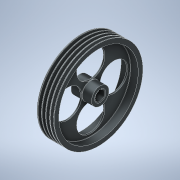
# Autodesk Inventor part: Polia Movida sem alivio de peso
Saved by Autodesk Inventor 2021 (Build 250183000, 183)
## iProperties
Created: 2021-03-22
Part Number: Polia Movida sem alivio de peso
Material: Iron, Cast
Document SubType Name: Modeling
Designer: mathe
Density: 7.15 g/cm^3
Appearance: Iron Gray
Mass: 8408.41 g
Surface Area: 3444.04 cm^2
Volume: 1176 cm^3
Author: mathe
Autodesk Inventor part; units mm, degrees
ref_plane "YZ Plane" through (0, 0, 0) normal (1, 0, 0) x (0, 1, 0)
ref_plane "XZ Plane" through (0, 0, 0) normal (0, 1, 0) x (-1, 0, 0)
ref_plane "XY Plane" through (0, 0, 0) normal (0, 0, 1) x (1, 0, 0)
sketch "Sketch1" plane through (0, 0, 0) normal (0, 0, 1) x (1, 0, 0)
  line L0 (68.9593, 13.1588) -> (64.9475, 24.81)
  line L1 (84.8393, 13.1588) -> (80.8275, 24.81)
  arc A0 (71.5582, 12.4844) -> (72.5037, 13.1588) centre (71.5582, 13.4844) ccw
  arc A1 (77.461, 25.4844) -> (76.5155, 24.81) centre (77.461, 24.4844) ccw
  line L2 (72.5037, 13.1588) -> (76.5155, 24.81)
  line L3 (56.6237, 13.1588) -> (60.6355, 24.81)
  arc A2 (82.7615, 30.4844) -> (83.7615, 31.4844) centre (82.7615, 31.4844) ccw
  arc A3 (82.7615, 30.4844) -> (83.7615, 31.4844) centre (82.7615, 31.4844) ccw
  arc A4 (80.8275, 24.81) -> (79.8819, 25.4844) centre (79.8819, 24.4844) ccw
  line L4 (69.9048, 12.4844) -> (71.5582, 12.4844)
  arc A5 (68.9593, 13.1588) -> (69.9048, 12.4844) centre (69.9048, 13.4844) ccw
  arc A6 (64.9475, 24.81) -> (64.0019, 25.4844) centre (64.0019, 24.4844) ccw
  line L5 (61.581, 25.4844) -> (64.0019, 25.4844)
  arc A7 (61.581, 25.4844) -> (60.6355, 24.81) centre (61.581, 24.4844) ccw
  arc A8 (55.6782, 12.4844) -> (56.6237, 13.1588) centre (55.6782, 13.4844) ccw
  line L6 (53.2615, 12.4844) -> (55.6782, 12.4844)
  line L7 (53.2615, 12.4844) -> (53.2615, 25.4844)
  line L8 (53.2615, 12.4844) -> (53.2615, 25.4844)
  line L9 (53.2615, 30.4844) -> (82.7615, 30.4844)
  line L10 (53.2615, 30.4844) -> (82.7615, 30.4844)
  line L11 (53.2615, 25.4844) -> (53.2615, 30.4844)
  line L12 (53.2615, 25.4844) -> (53.2615, 30.4844)
  line L13 (77.461, 25.4844) -> (79.8819, 25.4844)
  line L14 (83.7615, 149.9844) -> (83.7615, 31.4844)
  line L15 (89.7615, 149.9844) -> (89.7615, 31.4844)
  line L16 (83.7615, 149.9844) -> (83.7615, 31.4844)
  line L17 (89.7615, 149.9844) -> (89.7615, 31.4844)
  line L18 (68.9593, 356.81) -> (64.9475, 345.1588)
  line L19 (84.8393, 356.81) -> (80.8275, 345.1588)
  line L20 (88.3837, 356.81) -> (92.3955, 345.1588)
  arc A9 (72.5037, 356.81) -> (71.5582, 357.4844) centre (71.5582, 356.4844) ccw
  arc A10 (76.5155, 345.1588) -> (77.461, 344.4844) centre (77.461, 345.4844) ccw
  line L21 (53.2615, 339.4844) -> (82.7615, 339.4844)
  line L22 (53.2615, 339.4844) -> (82.7615, 339.4844)
  arc A11 (69.9048, 357.4844) -> (68.9593, 356.81) centre (69.9048, 356.4844) ccw
  line L23 (69.9048, 357.4844) -> (71.5582, 357.4844)
  line L24 (72.5037, 356.81) -> (76.5155, 345.1588)
  line L25 (77.461, 344.4844) -> (79.8819, 344.4844)
  arc A12 (79.8819, 344.4844) -> (80.8275, 345.1588) centre (79.8819, 345.4844) ccw
  arc A13 (85.7848, 357.4844) -> (84.8393, 356.81) centre (85.7848, 356.4844) ccw
  line L26 (85.7848, 357.4844) -> (87.4382, 357.4844)
  arc A14 (88.3837, 356.81) -> (87.4382, 357.4844) centre (87.4382, 356.4844) ccw
  arc A15 (83.7615, 338.4844) -> (82.7615, 339.4844) centre (82.7615, 338.4844) ccw
  arc A16 (90.7615, 339.4844) -> (89.7615, 338.4844) centre (90.7615, 338.4844) ccw
  arc A17 (90.7615, 339.4844) -> (89.7615, 338.4844) centre (90.7615, 338.4844) ccw
  arc A18 (83.7615, 338.4844) -> (82.7615, 339.4844) centre (82.7615, 338.4844) ccw
  line L27 (89.7615, 219.9844) -> (89.7615, 338.4844)
  line L28 (89.7615, 219.9844) -> (89.7615, 338.4844)
  line L29 (83.7615, 219.9844) -> (83.7615, 338.4844)
  line L30 (83.7615, 219.9844) -> (83.7615, 338.4844)
  arc A19 (82.7615, 218.9844) -> (83.7615, 219.9844) centre (82.7615, 219.9844) ccw
  arc A20 (82.7615, 218.9844) -> (83.7615, 219.9844) centre (82.7615, 219.9844) ccw
  arc A21 (89.7615, 219.9844) -> (90.7615, 218.9844) centre (90.7615, 219.9844) ccw
  arc A22 (89.7615, 219.9844) -> (90.7615, 218.9844) centre (90.7615, 219.9844) ccw
  line L31 (100.7193, 356.81) -> (96.7075, 345.1588)
  line L32 (104.2637, 356.81) -> (108.2755, 345.1588)
  line L33 (116.5993, 356.81) -> (112.5875, 345.1588)
  arc A23 (117.5448, 357.4844) -> (116.5993, 356.81) centre (117.5448, 356.4844) ccw
  line L34 (117.5448, 357.4844) -> (119.9615, 357.4844)
  arc A24 (101.6648, 357.4844) -> (100.7193, 356.81) centre (101.6648, 356.4844) ccw
  arc A25 (104.2637, 356.81) -> (103.3182, 357.4844) centre (103.3182, 356.4844) ccw
  line L35 (101.6648, 357.4844) -> (103.3182, 357.4844)
  arc A26 (108.2755, 345.1588) -> (109.221, 344.4844) centre (109.221, 345.4844) ccw
  arc A27 (111.6419, 344.4844) -> (112.5875, 345.1588) centre (111.6419, 345.4844) ccw
  line L36 (109.221, 344.4844) -> (111.6419, 344.4844)
  arc A28 (92.3955, 345.1588) -> (93.341, 344.4844) centre (93.341, 345.4844) ccw
  arc A29 (95.7619, 344.4844) -> (96.7075, 345.1588) centre (95.7619, 345.4844) ccw
  line L37 (93.341, 344.4844) -> (95.7619, 344.4844)
  line L38 (90.7615, 339.4844) -> (119.9615, 339.4844)
  line L39 (90.7615, 339.4844) -> (119.9615, 339.4844)
  line L40 (119.9615, 344.4844) -> (119.9615, 357.4844)
  line L41 (119.9615, 344.4844) -> (119.9615, 357.4844)
  line L42 (119.9615, 339.4844) -> (119.9615, 344.4844)
  line L43 (119.9615, 339.4844) -> (119.9615, 344.4844)
  line L44 (47.7615, 203.9844) -> (46.7615, 206.9844)
  line L45 (47.7615, 203.9844) -> (47.7615, 165.9844)
  line L46 (47.7615, 165.9844) -> (46.7615, 164.9844)
  line L47 (100.7193, 13.1588) -> (96.7075, 24.81)
  line L48 (88.3837, 13.1588) -> (92.3955, 24.81)
  line L49 (104.2637, 13.1588) -> (108.2755, 24.81)
  line L50 (116.5993, 13.1588) -> (112.5875, 24.81)
  arc A30 (116.5993, 13.1588) -> (117.5448, 12.4844) centre (117.5448, 13.4844) ccw
  line L51 (117.5448, 12.4844) -> (119.9615, 12.4844)
  arc A31 (100.7193, 13.1588) -> (101.6648, 12.4844) centre (101.6648, 13.4844) ccw
  arc A32 (103.3182, 12.4844) -> (104.2637, 13.1588) centre (103.3182, 13.4844) ccw
  line L52 (101.6648, 12.4844) -> (103.3182, 12.4844)
  arc A33 (84.8393, 13.1588) -> (85.7848, 12.4844) centre (85.7848, 13.4844) ccw
  line L53 (85.7848, 12.4844) -> (87.4382, 12.4844)
  arc A34 (87.4382, 12.4844) -> (88.3837, 13.1588) centre (87.4382, 13.4844) ccw
  arc A35 (89.7615, 31.4844) -> (90.7615, 30.4844) centre (90.7615, 31.4844) ccw
  arc A36 (89.7615, 31.4844) -> (90.7615, 30.4844) centre (90.7615, 31.4844) ccw
  arc A37 (93.341, 25.4844) -> (92.3955, 24.81) centre (93.341, 24.4844) ccw
  line L54 (93.341, 25.4844) -> (95.7619, 25.4844)
  arc A38 (96.7075, 24.81) -> (95.7619, 25.4844) centre (95.7619, 24.4844) ccw
  arc A39 (109.221, 25.4844) -> (108.2755, 24.81) centre (109.221, 24.4844) ccw
  line L55 (109.221, 25.4844) -> (111.6419, 25.4844)
  arc A40 (112.5875, 24.81) -> (111.6419, 25.4844) centre (111.6419, 24.4844) ccw
  line L56 (90.7615, 30.4844) -> (119.9615, 30.4844)
  line L57 (90.7615, 30.4844) -> (119.9615, 30.4844)
  line L58 (119.9615, 30.4844) -> (119.9615, 25.4844)
  line L59 (119.9615, 30.4844) -> (119.9615, 25.4844)
  line L60 (119.9615, 25.4844) -> (119.9615, 12.4844)
  line L61 (119.9615, 25.4844) -> (119.9615, 12.4844)
  arc A41 (64.0019, 344.4844) -> (64.9475, 345.1588) centre (64.0019, 345.4844) ccw
  line L62 (61.581, 344.4844) -> (64.0019, 344.4844)
  arc A42 (60.6355, 345.1588) -> (61.581, 344.4844) centre (61.581, 345.4844) ccw
  line L63 (53.2615, 344.4844) -> (53.2615, 339.4844)
  line L64 (53.2615, 344.4844) -> (53.2615, 339.4844)
  line L65 (56.6237, 356.81) -> (60.6355, 345.1588)
  arc A43 (56.6237, 356.81) -> (55.6782, 357.4844) centre (55.6782, 356.4844) ccw
  line L66 (53.2615, 357.4844) -> (55.6782, 357.4844)
  line L67 (53.2615, 357.4844) -> (53.2615, 344.4844)
  line L68 (53.2615, 357.4844) -> (53.2615, 344.4844)
  line L69 (46.7615, 218.9844) -> (46.7615, 150.9844)
  line L70 (82.7615, 218.9844) -> (46.7615, 218.9844)
  line L71 (82.7615, 218.9844) -> (46.7615, 218.9844)
  line L72 (82.7615, 150.9844) -> (46.7615, 150.9844)
  line L73 (82.7615, 150.9844) -> (46.7615, 150.9844)
  arc A44 (83.7615, 149.9844) -> (82.7615, 150.9844) centre (82.7615, 149.9844) ccw
  arc A45 (83.7615, 149.9844) -> (82.7615, 150.9844) centre (82.7615, 149.9844) ccw
  line L74 (125.7615, 165.9844) -> (47.7615, 165.9844)
  line L75 (47.7615, 203.9844) -> (125.7615, 203.9844)
  line L76 (46.7615, 206.9844) -> (126.7615, 206.9844)
  arc A46 (90.7615, 150.9844) -> (89.7615, 149.9844) centre (90.7615, 149.9844) ccw
  arc A47 (90.7615, 150.9844) -> (89.7615, 149.9844) centre (90.7615, 149.9844) ccw
  line L77 (125.7615, 203.9844) -> (126.7615, 206.9844)
  line L78 (126.7615, 218.9844) -> (90.7615, 218.9844)
  line L79 (126.7615, 218.9844) -> (90.7615, 218.9844)
  line L80 (125.7615, 165.9844) -> (125.7615, 203.9844)
  line L81 (126.7615, 150.9844) -> (90.7615, 150.9844)
  line L82 (126.7615, 150.9844) -> (90.7615, 150.9844)
  line L83 (125.7615, 165.9844) -> (126.7615, 164.9844)
  line L84 (126.7615, 150.9844) -> (126.7615, 218.9844)
  line L85 (130.2615, 184.9844) -> (43.5522, 184.9844)
  line L86 (343.2465, 11.6181) -> (339.2347, 23.2692)
  line L87 (359.1265, 11.6181) -> (355.1147, 23.2692)
  arc A48 (345.8454, 10.9436) -> (346.7909, 11.6181) centre (345.8454, 11.9436) ccw
  arc A49 (351.7483, 23.9436) -> (350.8027, 23.2692) centre (351.7483, 22.9436) ccw
  line L88 (346.7909, 11.6181) -> (350.8027, 23.2692)
  line L89 (330.9109, 11.6181) -> (334.9227, 23.2692)
  arc A50 (357.0487, 28.9436) -> (358.0487, 29.9436) centre (357.0487, 29.9436) ccw
  arc A51 (357.0487, 28.9436) -> (358.0487, 29.9436) centre (357.0487, 29.9436) ccw
  arc A52 (355.1147, 23.2692) -> (354.1692, 23.9436) centre (354.1692, 22.9436) ccw
  line L90 (344.192, 10.9436) -> (345.8454, 10.9436)
  arc A53 (343.2465, 11.6181) -> (344.192, 10.9436) centre (344.192, 11.9436) ccw
  arc A54 (339.2347, 23.2692) -> (338.2892, 23.9436) centre (338.2892, 22.9436) ccw
  line L91 (335.8683, 23.9436) -> (338.2892, 23.9436)
  arc A55 (335.8683, 23.9436) -> (334.9227, 23.2692) centre (335.8683, 22.9436) ccw
  arc A56 (329.9654, 10.9436) -> (330.9109, 11.6181) centre (329.9654, 11.9436) ccw
  line L92 (327.5487, 10.9436) -> (329.9654, 10.9436)
  line L93 (327.5487, 10.9436) -> (327.5487, 23.9436)
  line L94 (327.5487, 10.9436) -> (327.5487, 23.9436)
  line L95 (327.5487, 28.9436) -> (357.0487, 28.9436)
  line L96 (327.5487, 28.9436) -> (357.0487, 28.9436)
  line L97 (327.5487, 23.9436) -> (327.5487, 28.9436)
  line L98 (327.5487, 23.9436) -> (327.5487, 28.9436)
  line L99 (351.7483, 23.9436) -> (354.1692, 23.9436)
  line L100 (358.0487, 148.4436) -> (358.0487, 29.9436)
  line L101 (364.0487, 148.4436) -> (364.0487, 29.9436)
  line L102 (358.0487, 148.4436) -> (358.0487, 29.9436)
  line L103 (364.0487, 148.4436) -> (364.0487, 29.9436)
  line L104 (343.2465, 355.2692) -> (339.2347, 343.6181)
  line L105 (359.1265, 355.2692) -> (355.1147, 343.6181)
  line L106 (362.6709, 355.2692) -> (366.6827, 343.6181)
  arc A57 (346.7909, 355.2692) -> (345.8454, 355.9436) centre (345.8454, 354.9436) ccw
  arc A58 (350.8027, 343.6181) -> (351.7483, 342.9436) centre (351.7483, 343.9436) ccw
  line L107 (327.5487, 337.9436) -> (357.0487, 337.9436)
  line L108 (327.5487, 337.9436) -> (357.0487, 337.9436)
  arc A59 (344.192, 355.9436) -> (343.2465, 355.2692) centre (344.192, 354.9436) ccw
  line L109 (344.192, 355.9436) -> (345.8454, 355.9436)
  line L110 (346.7909, 355.2692) -> (350.8027, 343.6181)
  line L111 (351.7483, 342.9436) -> (354.1692, 342.9436)
  arc A60 (354.1692, 342.9436) -> (355.1147, 343.6181) centre (354.1692, 343.9436) ccw
  arc A61 (360.072, 355.9436) -> (359.1265, 355.2692) centre (360.072, 354.9436) ccw
  line L112 (360.072, 355.9436) -> (361.7254, 355.9436)
  arc A62 (362.6709, 355.2692) -> (361.7254, 355.9436) centre (361.7254, 354.9436) ccw
  arc A63 (358.0487, 336.9436) -> (357.0487, 337.9436) centre (357.0487, 336.9436) ccw
  arc A64 (365.0487, 337.9436) -> (364.0487, 336.9436) centre (365.0487, 336.9436) ccw
  arc A65 (365.0487, 337.9436) -> (364.0487, 336.9436) centre (365.0487, 336.9436) ccw
  arc A66 (358.0487, 336.9436) -> (357.0487, 337.9436) centre (357.0487, 336.9436) ccw
  line L113 (364.0487, 218.4436) -> (364.0487, 336.9436)
  line L114 (364.0487, 218.4436) -> (364.0487, 336.9436)
  line L115 (358.0487, 218.4436) -> (358.0487, 336.9436)
  line L116 (358.0487, 218.4436) -> (358.0487, 336.9436)
  arc A67 (357.0487, 217.4436) -> (358.0487, 218.4436) centre (357.0487, 218.4436) ccw
  arc A68 (357.0487, 217.4436) -> (358.0487, 218.4436) centre (357.0487, 218.4436) ccw
  arc A69 (364.0487, 218.4436) -> (365.0487, 217.4436) centre (365.0487, 218.4436) ccw
  arc A70 (364.0487, 218.4436) -> (365.0487, 217.4436) centre (365.0487, 218.4436) ccw
  line L117 (375.0065, 355.2692) -> (370.9947, 343.6181)
  line L118 (378.5509, 355.2692) -> (382.5627, 343.6181)
  line L119 (390.8865, 355.2692) -> (386.8747, 343.6181)
  arc A71 (391.832, 355.9436) -> (390.8865, 355.2692) centre (391.832, 354.9436) ccw
  line L120 (391.832, 355.9436) -> (394.2487, 355.9436)
  arc A72 (375.952, 355.9436) -> (375.0065, 355.2692) centre (375.952, 354.9436) ccw
  arc A73 (378.5509, 355.2692) -> (377.6054, 355.9436) centre (377.6054, 354.9436) ccw
  line L121 (375.952, 355.9436) -> (377.6054, 355.9436)
  arc A74 (382.5627, 343.6181) -> (383.5083, 342.9436) centre (383.5083, 343.9436) ccw
  arc A75 (385.9292, 342.9436) -> (386.8747, 343.6181) centre (385.9292, 343.9436) ccw
  line L122 (383.5083, 342.9436) -> (385.9292, 342.9436)
  arc A76 (366.6827, 343.6181) -> (367.6283, 342.9436) centre (367.6283, 343.9436) ccw
  arc A77 (370.0492, 342.9436) -> (370.9947, 343.6181) centre (370.0492, 343.9436) ccw
  line L123 (367.6283, 342.9436) -> (370.0492, 342.9436)
  line L124 (365.0487, 337.9436) -> (394.2487, 337.9436)
  line L125 (365.0487, 337.9436) -> (394.2487, 337.9436)
  line L126 (394.2487, 342.9436) -> (394.2487, 355.9436)
  line L127 (394.2487, 342.9436) -> (394.2487, 355.9436)
  line L128 (394.2487, 337.9436) -> (394.2487, 342.9436)
  line L129 (394.2487, 337.9436) -> (394.2487, 342.9436)
  line L130 (322.0487, 202.4436) -> (321.0487, 205.4436)
  line L131 (322.0487, 202.4436) -> (322.0487, 164.4436)
  line L132 (322.0487, 164.4436) -> (321.0487, 163.4436)
  line L133 (375.0065, 11.6181) -> (370.9947, 23.2692)
  line L134 (362.6709, 11.6181) -> (366.6827, 23.2692)
  line L135 (378.5509, 11.6181) -> (382.5627, 23.2692)
  line L136 (390.8865, 11.6181) -> (386.8747, 23.2692)
  arc A78 (390.8865, 11.6181) -> (391.832, 10.9436) centre (391.832, 11.9436) ccw
  line L137 (391.832, 10.9436) -> (394.2487, 10.9436)
  arc A79 (375.0065, 11.6181) -> (375.952, 10.9436) centre (375.952, 11.9436) ccw
  arc A80 (377.6054, 10.9436) -> (378.5509, 11.6181) centre (377.6054, 11.9436) ccw
  line L138 (375.952, 10.9436) -> (377.6054, 10.9436)
  arc A81 (359.1265, 11.6181) -> (360.072, 10.9436) centre (360.072, 11.9436) ccw
  line L139 (360.072, 10.9436) -> (361.7254, 10.9436)
  arc A82 (361.7254, 10.9436) -> (362.6709, 11.6181) centre (361.7254, 11.9436) ccw
  arc A83 (364.0487, 29.9436) -> (365.0487, 28.9436) centre (365.0487, 29.9436) ccw
  arc A84 (364.0487, 29.9436) -> (365.0487, 28.9436) centre (365.0487, 29.9436) ccw
  arc A85 (367.6283, 23.9436) -> (366.6827, 23.2692) centre (367.6283, 22.9436) ccw
  line L140 (367.6283, 23.9436) -> (370.0492, 23.9436)
  arc A86 (370.9947, 23.2692) -> (370.0492, 23.9436) centre (370.0492, 22.9436) ccw
  arc A87 (383.5083, 23.9436) -> (382.5627, 23.2692) centre (383.5083, 22.9436) ccw
  line L141 (383.5083, 23.9436) -> (385.9292, 23.9436)
  arc A88 (386.8747, 23.2692) -> (385.9292, 23.9436) centre (385.9292, 22.9436) ccw
  line L142 (365.0487, 28.9436) -> (394.2487, 28.9436)
  line L143 (365.0487, 28.9436) -> (394.2487, 28.9436)
  line L144 (394.2487, 28.9436) -> (394.2487, 23.9436)
  line L145 (394.2487, 28.9436) -> (394.2487, 23.9436)
  line L146 (394.2487, 23.9436) -> (394.2487, 10.9436)
  line L147 (394.2487, 23.9436) -> (394.2487, 10.9436)
  arc A89 (338.2892, 342.9436) -> (339.2347, 343.6181) centre (338.2892, 343.9436) ccw
  line L148 (335.8683, 342.9436) -> (338.2892, 342.9436)
  arc A90 (334.9227, 343.6181) -> (335.8683, 342.9436) centre (335.8683, 343.9436) ccw
  line L149 (327.5487, 342.9436) -> (327.5487, 337.9436)
  line L150 (327.5487, 342.9436) -> (327.5487, 337.9436)
  line L151 (330.9109, 355.2692) -> (334.9227, 343.6181)
  arc A91 (330.9109, 355.2692) -> (329.9654, 355.9436) centre (329.9654, 354.9436) ccw
  line L152 (327.5487, 355.9436) -> (329.9654, 355.9436)
  line L153 (327.5487, 355.9436) -> (327.5487, 342.9436)
  line L154 (327.5487, 355.9436) -> (327.5487, 342.9436)
  line L155 (321.0487, 217.4436) -> (321.0487, 149.4436)
  line L156 (357.0487, 217.4436) -> (321.0487, 217.4436)
  line L157 (357.0487, 217.4436) -> (321.0487, 217.4436)
  line L158 (357.0487, 149.4436) -> (321.0487, 149.4436)
  line L159 (357.0487, 149.4436) -> (321.0487, 149.4436)
  arc A92 (358.0487, 148.4436) -> (357.0487, 149.4436) centre (357.0487, 148.4436) ccw
  arc A93 (358.0487, 148.4436) -> (357.0487, 149.4436) centre (357.0487, 148.4436) ccw
  line L160 (400.0487, 164.4436) -> (322.0487, 164.4436)
  line L161 (322.0487, 202.4436) -> (400.0487, 202.4436)
  line L162 (321.0487, 205.4436) -> (401.0487, 205.4436)
  arc A94 (365.0487, 149.4436) -> (364.0487, 148.4436) centre (365.0487, 148.4436) ccw
  arc A95 (365.0487, 149.4436) -> (364.0487, 148.4436) centre (365.0487, 148.4436) ccw
  line L163 (400.0487, 202.4436) -> (401.0487, 205.4436)
  line L164 (401.0487, 217.4436) -> (365.0487, 217.4436)
  line L165 (401.0487, 217.4436) -> (365.0487, 217.4436)
  line L166 (400.0487, 164.4436) -> (400.0487, 202.4436)
  line L167 (401.0487, 149.4436) -> (365.0487, 149.4436)
  line L168 (401.0487, 149.4436) -> (365.0487, 149.4436)
  line L169 (400.0487, 164.4436) -> (401.0487, 163.4436)
  line L170 (401.0487, 149.4436) -> (401.0487, 217.4436)
  line L171 (404.5487, 183.4436) -> (317.8394, 183.4436)
  point P0 (0, 0)
  dimension "d1" = 80
  dimension "d3" = 1
  dimension "d5" = 38
  dimension "d7" = 68
  dimension "d9" = 38
  dimension "d11" = 13
  dimension "d13" = 80
  dimension "d15" = 1
  dimension "d17" = 38
  dimension "d19" = 68
  dimension "d21" = 38
  dimension "d23" = 13
  constraints: 344 end point, 192 point on circle, 96 centre point, 8 point on line
  measures "d1" distance of L69.end L81.start
  measures "d3" radius of A45
  measures "d5" angle of L18 L65
  measures "d7" distance of L69.start L69.end
  measures "d9" distance of L44.start L45.end
  measures "d11" distance from line of L62 L66.start
  measures "d13" distance of L155.end L167.start
  measures "d15" radius of A93
  measures "d17" angle of L104 L151
  measures "d19" distance of L155.start L155.end
  measures "d21" distance of L130.start L131.end
  measures "d23" distance from line of L148 L152.start
revolve "Revolution1" add sketch "Sketch1" angle 360 about axis through (130.2615, 184.9844, 0) along (-1, 0, 0) contours L76 L77 L75 L44 | L69 L70 A19 L29 A15 L21 L63 L67 L66 A43 L65 A42 L62 A41 L18 A11 L23 A9 L24 A10 L25 A12 L19 A13 L26 A14 L20 A28 L37 A29 L31 A24 L35 A25 L32 A26 L36 A27 L33 A23 L34 L40 L42 L38 A16 L27 A21 L78 L84 L76
sketch "Sketch2" plane through (46.7615, 184.9844, 0) normal (-1, 0, 0) x (0, 0, 1)
  circle A0 centre (0, 0) radius 19 projected
  line L0 (0, 19) -> (0, 22.2)
  line L1 (0, 22.2) -> (5, 22.2)
  line L2 (5, 22.2) -> (5, 18.3303)
  line L3 (0, 22.2) -> (-5, 22.2)
  line L4 (-5, 22.2) -> (-5, 18.3303)
  point P0 (0, -184.9844)
  dimension "d25" = 3.2
  dimension "d26" = 5
  dimension "d27" = 5
  constraints: 10 end point, 3 point on circle, 2 perpendicular, 1 horizontal, 1 vertical
  measures "d25" distance of L0.start L0.end
  measures "d26" distance of L0.end L1.end
  measures "d27" distance of L0.end L3.end
extrude "Extrusion1" cut sketch "Sketch2" against normal through all contours A0 L0 L1 L2 | L4 L3 L0 A0
sketch "Sketch3" plane through (46.7615, 184.9844, 0) normal (-1, 0, 0) x (0, 0, 1)
  circle A0 centre (0, 0) radius 34 projected
  circle A1 centre (0, 0) radius 90
  line L0 (0, 0) -> (111, 0)
  circle A2 centre (90, 0) radius 55
  circle A3 centre (0, 90) radius 55
  circle A4 centre (-90, 0) radius 55
  circle A5 centre (0, -90) radius 55
  point P0 (0, -184.9844)
  dimension "d30" = 180
  dimension "d31" = 110
  dimension "d34" = 360
  constraints: 4 centre point, 2 end point, 1 coincident, 1 horizontal, 1 horizontal alignment, 1 point on line, 11 other
  measures "d31" diameter of A2
extrude "Extrusion2" cut sketch "Sketch3" against normal blind 1000 contours A2 A1 L0 | L0 A1 A2 | A1 A2 | A3 A1 | A1 A3 | A5 A1 | A1 A5 | A4 A1 | A1 A4
body "Solid1"
